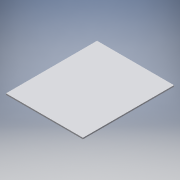
# Autodesk Inventor part: PitchingMachineBase
Saved by Autodesk Inventor 2016 SP1 (Build 200210100, 210)
## iProperties
Created: 2016-01-12
Part Number: PitchingMachineBase
Material: Aluminum 6061
Document SubType Name: Modeling
Designer: steele
Density: 2.7 g/cm^3
Appearance: Aluminum - Flat
Author: steele
Autodesk Inventor part; units mm, degrees
ref_plane "YZ Plane" through (0, 0, 0) normal (1, 0, 0) x (0, 1, 0)
ref_plane "XZ Plane" through (0, 0, 0) normal (0, 1, 0) x (-1, 0, 0)
ref_plane "XY Plane" through (0, 0, 0) normal (0, 0, 1) x (1, 0, 0)
sketch "Sketch1" plane through (0, 0, 0) normal (0, 1, 0) x (-1, 0, 0)
  line L0 (190.5, 225.425) -> (-190.5, 225.425)
  line L1 (-190.5, 225.425) -> (-190.5, -225.425)
  line L2 (-190.5, -225.425) -> (190.5, -225.425)
  line L3 (190.5, -225.425) -> (190.5, 225.425)
  line L4 (190.5, 225.425) -> (-190.5, -225.425) construction
  line L5 (-190.5, 225.425) -> (190.5, -225.425) construction
  point P0 (0, 0)
  dimension "d0" = 381
  dimension "d1" = 450.85
  constraints: 12 end point, 2 midpoint, 2 parallel, 1 horizontal, 1 perpendicular
  measures "d0" distance of L0.start L0.end
  measures "d1" distance of L2.end L0.start
extrude "Extrusion1" add sketch "Sketch1" against normal blind 6.35
equation "\"d0\" = pitchingMachineBaseLength"
equation "\"d1\" = pitchingMachineBaseWidth"
equation "\"d2\" = pitchingMachineBaseDepth"
equation "\"pitchingMachineBaseWidth\" = 450.85"
equation "\"pitchingMachineBaseLength\" = 381"
equation "\"pitchingMachineBaseDepth\" = 6.35"
body "Solid1"
